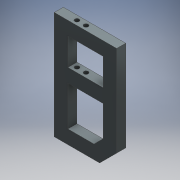
# Autodesk Inventor part: chassi_back_right
Saved by Autodesk Inventor 2016 (Build 200138000, 138)
## iProperties
Created: 2017-01-03
Part Number: chassi_back_right
Material: Generic
Document SubType Name: Modeling
Designer: hesaon
Density: 1 g/cm^3
Appearance: Default
Author: hesaon
Autodesk Inventor part; units mm, degrees
ref_plane "YZ Plane" through (0, 0, 0) normal (1, 0, 0) x (0, 1, 0)
ref_plane "XZ Plane" through (0, 0, 0) normal (0, 1, 0) x (-1, 0, 0)
ref_plane "XY Plane" through (0, 0, 0) normal (0, 0, 1) x (1, 0, 0)
sketch "Sketch1" plane through (0, 0, 0) normal (0, 1, 0) x (-1, 0, 0)
  line L0 (0, 142.5) -> (0, 0)
  line L1 (0, 142.5) -> (-82.5, 142.5)
  line L2 (0, 0) -> (-60, 0)
  line L3 (-60, 0) -> (-82.5, 22.5)
  line L4 (-82.5, 142.5) -> (-82.5, 22.5)
  line L5 (-18, 18) -> (-52.5442, 18)
  line L6 (-64.5, 124.5) -> (-18, 124.5)
  line L7 (-18, 88.5) -> (-64.5, 88.5)
  line L8 (-18, 70.5) -> (-64.5, 70.5)
  line L9 (-18, 124.5) -> (-18, 88.5)
  line L10 (-18, 70.5) -> (-18, 18)
  line L11 (-64.5, 29.9558) -> (-64.5, 70.5)
  line L12 (-64.5, 88.5) -> (-64.5, 124.5)
  line L13 (-52.5442, 18) -> (-64.5, 29.9558)
  dimension "d1" = 142.5
  dimension "d3" = 82.5
  dimension "d4" = 60
  dimension "d5" = 135
  dimension "d6" = 120
  dimension "d8" = 18
  dimension "d9" = 18
  dimension "d15" = 88.5
  dimension "d16" = 18
  dimension "d17" = 18
  dimension "d18" = 18
  dimension "d19" = 18
  dimension "d20" = 18
  dimension "d21" = 18
  constraints: 28 end point, 6 perpendicular, 3 vertical, 2 horizontal, 2 parallel, 1 coincident
  measures "d1" distance of L0.end L0.start
  measures "d3" distance of L0.start L1.end
  measures "d4" distance of L0.end L2.end
  measures "d5" angle of L2 L3
  measures "d6" distance of L3.end L1.end
  measures "d8" distance between parallel lines of L1 L6
  measures "d9" distance between parallel lines of L2 L5
  measures "d15" distance between parallel lines of L2 L7
  measures "d16" distance between parallel lines of L8 L7
  measures "d17" distance of L8.end L7.end
  measures "d18" distance from line of L0 L6.end
  measures "d19" distance between parallel lines of L0 L10
  measures "d20" distance between parallel lines of L4 L12
  measures "d21" distance between parallel lines of L3 L13
extrude "Extrusion2" add sketch "Sketch1" along normal blind 12
sketch "Sketch3" plane through (0, 0, 142.5) normal (0, 0, 1) x (1, 0, 0)
  line L0 (52.5442, 0) -> (52.5442, 12) projected
  line L1 (18, 0) -> (18, 12) projected
  circle A0 centre (24, 6) radius 2.85
  line L2 (82.5, 0) -> (0, 0) projected
  circle A1 centre (36, 6) radius 2.85
  dimension "d24" = 5.7
  dimension "d25" = 6
  dimension "d26" = 6
  dimension "d27" = 5.7
  dimension "d28" = 12
  dimension "d29" = 6
  constraints: 2 centre point
  measures "d24" diameter of A0
  measures "d25" distance from line of L1 A0.centre
  measures "d26" distance from line of A0.centre L2
  measures "d27" diameter of A1
  measures "d28" distance of A0.centre A1.centre
  measures "d29" distance from line of L2 A1.centre
extrude "Extrusion3" cut sketch "Sketch3" against normal blind 72
sketch "Sketch4" plane through (64.5, 0, 70.5) normal (0, 0, -1) x (-1, 0, 0)
  circle A0 centre (40.5, 6) radius 2.85 projected
  circle A1 centre (28.5, 6) radius 2.85 projected
  circle A2 centre (40.5, 6) radius 2.85 projected
  line L0 (37.4978, 0.8) -> (34.4956, 6)
  line L1 (34.4956, 6) -> (37.4978, 11.2)
  line L2 (37.4978, 11.2) -> (43.5022, 11.2)
  line L3 (43.5022, 11.2) -> (46.5044, 6)
  line L4 (46.5044, 6) -> (43.5022, 0.8)
  line L5 (43.5022, 0.8) -> (37.4978, 0.8)
  line L6 (25.442, 0.8322) -> (22.4956, 6.0644)
  line L7 (22.4956, 6.0644) -> (25.5535, 11.2322)
  line L8 (25.5535, 11.2322) -> (31.558, 11.1678)
  line L9 (31.558, 11.1678) -> (34.5044, 5.9356)
  line L10 (34.5044, 5.9356) -> (31.4465, 0.7678)
  line L11 (31.4465, 0.7678) -> (25.442, 0.8322)
  line L12 (0, 0) -> (46.5, 0) projected
  point P0 (64.5, 0)
  point P1 (28.4442, 0.8)
  dimension "d32" = 10.4
  constraints: 24 end point, 2 coincident, 1 midpoint, 1 parallel, 1 point on line, 26 other
  measures "d32" distance between parallel lines of L5 L2
extrude "Extrusion4" cut sketch "Sketch4" against normal blind 5
body "Solid2"
